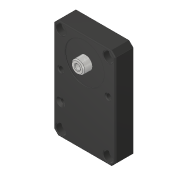
# Autodesk Inventor part: XM430_HOUSING_TOP
Saved by Autodesk Inventor 2019.4 (Build 234330000, 330)
## iProperties
Created: 2019-10-08
Part Number: XM430_HOUSING_TOP
Material: 一般
Document SubType Name: Modeling
Designer: y6tada
Density: 1 g/cm^3
Appearance: 滑らか - 黒
Author: y6tada
Autodesk Inventor part; units mm, degrees
ref_plane "YZ Plane" through (0, 0, 0) normal (1, 0, 0) x (0, 1, 0)
ref_plane "XZ Plane" through (0, 0, 0) normal (0, 1, 0) x (-1, 0, 0)
ref_plane "XY Plane" through (0, 0, 0) normal (0, 0, 1) x (1, 0, 0)
sketch "スケッチ1" plane through (0, 0, 0) normal (0, 0, 1) x (1, 0, 0)
  line L0 (-12.25, 11.25) -> (12.25, 11.25)
  line L1 (14.25, 9.25) -> (14.25, -33.25)
  line L2 (12.25, -35.25) -> (-12.25, -35.25)
  line L3 (-14.25, -33.25) -> (-14.25, 9.25)
  circle A0 centre (11, 8) radius 1.25
  circle A1 centre (11, -8) radius 1.25
  circle A2 centre (11, -32) radius 1.25
  line L4 (0, 0) -> (0, 13.0678) construction
  circle A3 centre (-11, 8) radius 1.25
  circle A4 centre (-11, -8) radius 1.25
  circle A5 centre (-11, -32) radius 1.25
  line L5 (-26.5405, 0) -> (16.6243, 0) construction
  line L6 (11, 8) -> (11, -8) construction
  line L7 (11, -8) -> (11, -32) construction
  circle A6 centre (-11, -21.05) radius 1
  line L8 (-11, -21.05) -> (-11, -32) construction
  line L9 (-14.25, 9.25) -> (-12.25, 11.25)
  line L10 (12.25, 11.25) -> (14.25, 9.25)
  line L11 (12.25, -35.25) -> (14.25, -33.25)
  line L12 (-14.25, -33.25) -> (-12.25, -35.25)
  circle A7 centre (0, 0) radius 3.2
  point P0 (-14.25, 11.25)
  point P1 (14.25, -35.25)
  point P2 (14.25, 11.25)
  point P3 (-14.25, -35.25)
  dimension "d0" = 2.5
  dimension "d1" = 28.5
  dimension "d3" = 46.5
  dimension "d4" = 8
  dimension "d5" = 8
  dimension "d6" = 22
  dimension "d7" = 40
  dimension "d8" = 2
  dimension "d9" = 14.2
  dimension "d10" = 11.25
  dimension "d11" = 2
  dimension "d12" = 2
  dimension "d13" = 2
  dimension "d14" = 2
  dimension "d15" = 2
  dimension "d16" = 2
  dimension "d17" = 2
  dimension "d18" = 2
  dimension "d41" = 6.4
  constraints: 26 end point, 9 point on line, 8 centre point, 3 symmetric about line, 3 vertical, 2 coincident, 2 equal radius, 2 horizontal, 2 parallel, 1 collinear, 1 perpendicular, 4 other
  measures "d0" diameter of A0
  measures "d1" distance between parallel lines of L1 L3
  measures "d3" distance between parallel lines of L2 L0
  measures "d4" distance from line of L5 L6.start
  measures "d5" distance from line of L5 L6.end
  measures "d6" distance of L6.start A3.centre
  measures "d7" distance of L7.end L6.start
  measures "d8" diameter of A6
  measures "d9" distance from line of L2 L8.start
  measures "d10" distance between parallel lines of L5 L0
  measures "d11" distance of L3.end point (-14.25, 11.25)
  measures "d12" distance of L0.start point (-14.25, 11.25)
  measures "d13" distance of L0.end point (14.25, 11.25)
  measures "d14" distance of L1.start point (14.25, 11.25)
  measures "d15" distance of L2.start point (14.25, -35.25)
  measures "d16" distance of L1.end point (14.25, -35.25)
  measures "d17" distance of L3.start point (-14.25, -35.25)
  measures "d18" distance of L2.end point (-14.25, -35.25)
  measures "d41" diameter of A7
extrude "押し出し1" add sketch "スケッチ1" against normal blind 8.5
chamfer "面取り1" distance 1.1 angle 45 1 edges at (-12, -21.05, 0)
sketch "スケッチ2" plane through (0, 0, 0) normal (0, 0, 1) x (1, 0, 0)
  circle A0 centre (-11, 8) radius 2.4
  circle A1 centre (11, 8) radius 2.4
  circle A2 centre (11, -32) radius 2.4
  circle A3 centre (-11, -32) radius 2.4
  circle A4 centre (-11, 8) radius 1.25 construction
  circle A5 centre (11, 8) radius 1.25 construction
  circle A6 centre (11, -32) radius 1.25 construction
  circle A7 centre (-11, -32) radius 1.25 construction
  point P0 (0, 0)
  dimension "d25" = 4.8
  constraints: 4 centre point, 4 coincident, 4 concentric, 3 equal radius
  measures "d25" diameter of A1
extrude "押し出し2" cut sketch "スケッチ2" against normal blind 2.8
sketch "スケッチ3" plane through (0, 0, 0) normal (0, 0, 1) x (1, 0, 0)
  circle A0 centre (0, 0) radius 9
  dimension "d40" = 18
  constraints: 1 centre point, 1 coincident
  measures "d40" diameter of A0
extrude "押し出し3" cut sketch "スケッチ3" against normal blind 0.5
chamfer "面取り2" distance 0.4 angle 45 10 edges at (-14.25, -12, 0) (-13.25, 10.25, 0) (0, 11.25, 0) (13.25, 10.25, 0) (14.25, -12, 0) (13.25, -34.25, 0) (0, -35.25, 0) (-13.25, -34.25, 0) (-12.25, -8, 0) (9.75, -8, 0)
chamfer "面取り3" distance 0.2 angle 45 13 edges at (-13.4, 8, 0) (8.6, 8, 0) (-9, 0, 0) (8.6, -32, 0) (-13.4, -32, 0) (-14.25, -12, -8.5) (-13.25, -34.25, -8.5) (0, -35.25, -8.5) (13.25, -34.25, -8.5) (14.25, -12, -8.5) (13.25, 10.25, -8.5) (0, 11.25, -8.5) (-13.25, 10.25, -8.5)
sketch "スケッチ5" plane through (0, 0, 0) normal (0, 1, 0) x (-1, 0, 0)
  line L0 (-1.25, -8.5) -> (-3, -8.5)
  line L1 (-3, -8.5) -> (-3, 2.85)
  line L2 (-2.5, 3.35) -> (-1.5, 3.35)
  line L3 (-1.25, 3.1) -> (-1.25, -8.5)
  line L4 (12.1672, -8.5) -> (-12.1672, -8.5) construction
  line L5 (-12.0843, 0) -> (12.0843, 0) construction
  line L6 (0, 0) -> (0, -12.5423) construction
  line L7 (-3, 2.85) -> (-2.5, 3.35)
  line L8 (-1.5, 3.35) -> (-1.25, 3.1)
  point P0 (-3, 3.35)
  point P1 (-1.25, 3.35)
  dimension "d42" = 2.5
  dimension "d43" = 6
  dimension "d44" = 3.35
  dimension "d45" = 0.5
  dimension "d46" = 0.5
  dimension "d47" = 0.25
  dimension "d48" = 0.25
  constraints: 14 end point, 4 point on line, 2 parallel, 1 collinear, 1 horizontal, 1 perpendicular, 1 vertical
  measures "d42" diameter of L3 L6
  measures "d43" diameter of L1 L6
  measures "d44" distance between parallel lines of L5 L2
  measures "d45" distance of L1.end point (-3, 3.35)
  measures "d46" distance of L2.start point (-3, 3.35)
  measures "d47" distance of L2.end point (-1.25, 3.35)
  measures "d48" distance of L3.start point (-1.25, 3.35)
revolve "回転1" add sketch "スケッチ5" angle 360 about axis through (0, 0, 0) along (0, 0, -1)
equation "\"d12\" = d11"
equation "\"d13\" = d11"
equation "\"d14\" = d13"
equation "\"d15\" = d11"
equation "\"d16\" = d15"
equation "\"d17\" = d11"
equation "\"d18\" = d17"
equation "\"d46\" = d45"
equation "\"d48\" = d47"
